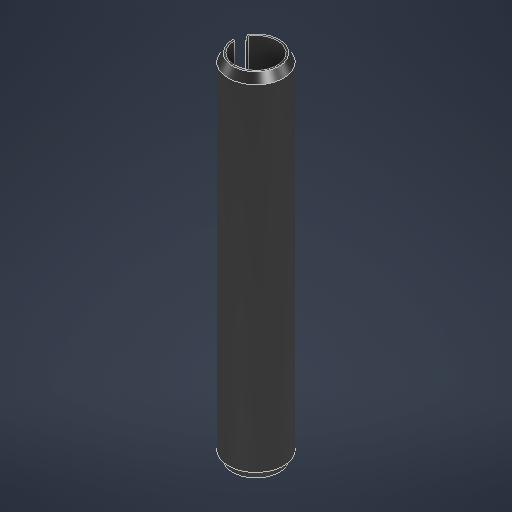
# Autodesk Inventor part: Part9
Saved by Autodesk Inventor 2026 (Build 300175000, 175)
## iProperties
Created: 2026-03-22
Part Number: Part9
Material: Generic
Document SubType Name: Modeling
Designer: Mlinč
Density: 1 g/cm^3
Appearance: Default
Author: Mlinč
Autodesk Inventor part; units mm, degrees
ref_plane "YZ Plane" through (0, 0, 0) normal (1, 0, 0) x (0, 1, 0)
ref_plane "XZ Plane" through (0, 0, 0) normal (0, 1, 0) x (-1, 0, 0)
ref_plane "XY Plane" through (0, 0, 0) normal (0, 0, 1) x (1, 0, 0)
sketch "Sketch1" plane through (0, 0, 0) normal (0, 0, 1) x (1, 0, 0)
  line L0 (-2.3, 0) -> (-3, 0)
  line L1 (-3, 0) -> (-3, 38)
  line L2 (-3, 38) -> (-2.3, 38)
  line L3 (-2.3, 38) -> (-2.3, 0)
  line L4 (0, 0) -> (0, 38)
  point P0 (-2.65, 38)
  point P1 (-2.65, 0)
  dimension "d0" = 0.7
  dimension "d1" = 6
  dimension "d2" = 38
  constraints: 10 end point, 2 horizontal alignment, 2 midpoint, 2 parallel, 1 horizontal, 1 perpendicular, 1 vertical
  measures "d0" distance of L1.end L2.end
  measures "d1" diameter of L1 L4
  measures "d2" distance of L4.start L4.end
revolve "Revolution1" add sketch "Sketch1" angle 330 about axis through (0, 0, 0) along (0, 1, 0)
chamfer "Chamfer1" distance 0.5 angle 60 1 edges at (2.8978, 38, 0.7765) measured on face at (-0.4754, 38, -2.7069)
chamfer "Chamfer2" distance 0.5 angle 60 1 edges at (2.8978, 0, 0.7765) measured on face at (1.8107, 0, -2.0675)
body "Solid1"
